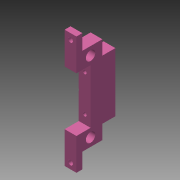
# Autodesk Inventor part: Part9
Saved by Autodesk Inventor 2015 (Build 190159000, 159)
## iProperties
Created: 2015-07-07
Part Number: Part9
Material: ABS Plastic
Document SubType Name: Modeling
Designer: hp
Density: 1.06 g/cm^3
Appearance: Smooth - Dark Sea Green
Author: hp
Autodesk Inventor part; units mm, degrees
ref_plane "YZ Plane" through (0, 0, 0) normal (1, 0, 0) x (0, 1, 0)
ref_plane "XZ Plane" through (0, 0, 0) normal (0, 1, 0) x (-1, 0, 0)
ref_plane "XY Plane" through (0, 0, 0) normal (0, 0, 1) x (1, 0, 0)
sketch "Sketch1" plane through (0, 0, 0) normal (1, 0, 0) x (0, 1, 0)
  line L0 (0, 50) -> (0, 23)
  line L1 (0, 23) -> (12, 23)
  line L2 (12, 23) -> (12, -23)
  line L3 (12, -23) -> (0, -23)
  line L4 (0, -23) -> (0, -50)
  line L5 (0, -50) -> (5, -50)
  line L6 (5, -50) -> (5, -37)
  line L7 (5, -37) -> (22, -37)
  line L8 (22, -37) -> (22, -25)
  line L9 (22, -25) -> (33, -25)
  line L10 (33, -25) -> (33, 25)
  line L11 (33, 25) -> (22, 25)
  line L12 (22, 25) -> (22, 37)
  line L13 (22, 37) -> (5, 37)
  line L14 (5, 37) -> (5, 50)
  line L15 (5, 50) -> (0, 50)
  circle A0 centre (12, 30) radius 4
  circle A1 centre (12, -30) radius 4
  point P0 (0, 0)
  point P1 (12, 0)
  dimension "d0" = 100
  dimension "d1" = 46
  dimension "d2" = 27
  dimension "d3" = 5
  dimension "d4" = 17
  dimension "d5" = 13
  dimension "d6" = 12
  dimension "d7" = 11
  dimension "d8" = 12
  dimension "d9" = 8
  dimension "d10" = 30
  dimension "d11" = 30
  dimension "d12" = 12
  constraints: 32 end point, 12 perpendicular, 6 point on line, 2 centre point, 2 collinear, 2 vertical alignment, 1 equal radius, 1 horizontal alignment, 1 midpoint, 1 vertical
  measures "d0" distance between parallel lines of L5 L15
  measures "d1" distance of L1.end L2.end
  measures "d2" distance of L3.end L4.end
  measures "d3" distance of L4.end L5.end
  measures "d4" distance of L6.end L7.end
  measures "d5" distance of L5.end L6.end
  measures "d6" distance of L7.end L8.end
  measures "d7" distance of L8.end L9.end
  measures "d8" distance of L2.end L3.end
  measures "d9" diameter of A0
  measures "d10" vertical distance of point (0, 0) A0.centre
  measures "d11" vertical distance of point (0, 0) A1.centre
  measures "d12" distance from line of L0 A0.centre
extrude "Extrusion1" add sketch "Sketch1" along normal blind 10
sketch "Sketch2" plane through (0, 0, 23) normal (0, -1, 0) x (1, 0, 0)
  circle A0 centre (5, 22) radius 2
  circle A1 centre (5, -7.5) radius 1.6
  circle A2 centre (5, -38.5) radius 1.6
  circle A3 centre (5, -68) radius 2
  line L0 (0, 27) -> (10, 27) projected
  point P0 (0, -23)
  point P1 (5, 27)
  dimension "d15" = 4
  dimension "d16" = 3.2
  dimension "d17" = 15.5
  dimension "d18" = 15.5
  dimension "d19" = 90
  dimension "d20" = 45
  constraints: 4 centre point, 4 vertical alignment, 2 equal radius, 1 midpoint
  measures "d15" diameter of A0
  measures "d16" diameter of A1
  measures "d17" vertical distance of point (0, -23) A1.centre
  measures "d18" vertical distance of point (0, -23) A2.centre
  measures "d19" distance of A3.centre A0.centre
  measures "d20" vertical distance of point (0, -23) A0.centre
extrude "Extrusion2" cut sketch "Sketch2" against normal through all
sketch "Sketch3" plane through (0, 33, 25) normal (0, 1, 0) x (1, 0, 0)
  line L0 (0.3, 25) -> (0, 25.72)
  line L1 (0, 50) -> (0, 0) projected
  line L2 (0, 24.28) -> (0.3, 25)
  point P0 (0, 25)
  point P1 (0, 25)
  dimension "d23" = 0.72
  dimension "d24" = 0.3
  dimension "d25" = 0.72
  constraints: 4 end point, 2 point on line, 1 horizontal alignment, 1 midpoint
  measures "d23" distance of L0.end point (0, 25)
  measures "d24" horizontal distance of L0.start L0.end
  measures "d25" distance of point (0, 25) L2.start
extrude "Extrusion3" cut sketch "Sketch3" against normal up to next
equation "\"d11\" = d10"
equation "\"d18\" = d17"
equation "\"d21\" = d18"
body "Solid1"
